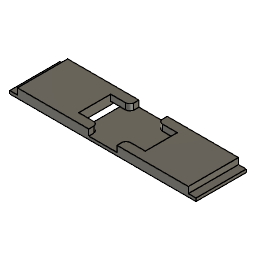
Canal - middle plate v6 (Autodesk Fusion 360 design; units mm, degrees)
Autodesk Fusion 360 part; units mm, degrees
sketch "Esquisse1" plane through (0, 0, 0) normal (0, 0, 1) x (1, 0, 0)
  line L0 (9.4, 40) -> (70, 40)
  line L1 (70, 40) -> (70, 23.65)
  line L2 (70, 23.65) -> (9.4, 23.65)
  line L3 (9.4, 23.65) -> (9.4, 40)
  dimension "d1" = 60.6
  dimension "d2" = 16.35
  constraint horizontal L0
  constraint vertical L1
  constraint horizontal L2
  constraint vertical L3
  measures "d1" distance of L1 L3
  measures "d2" distance of L0 L2
extrude "Extrusion1" add sketch "Esquisse1" along normal blind 3
sketch "Esquisse2" plane through (0, 0, 0) normal (0, 0, -1) x (1, 0, 0)
  line L0 (70, -23.65) -> (9.4, -23.65)
  line L1 (9.4, -23.65) -> (9.4, -40)
  line L2 (9.4, -40) -> (70, -40)
  line L3 (70, -40) -> (70, -23.65)
  line L4 (17.1, -25.55) -> (22.3, -25.55)
  line L5 (22.3, -25.55) -> (22.3, -27.75)
  line L6 (22.3, -27.75) -> (17.1, -27.75)
  line L7 (17.1, -27.75) -> (17.1, -25.55)
  line L8 (19.7, -25.55) -> (19.7, -27.75) construction
  line L9 (39.7, -23.65) -> (39.7, -40) construction
  line L10 (57.1, -25.55) -> (57.1, -27.75)
  line L11 (62.3, -25.55) -> (57.1, -25.55)
  line L12 (62.3, -27.75) -> (62.3, -25.55)
  line L13 (57.1, -27.75) -> (62.3, -27.75)
  line L14 (9.4, -31.825) -> (70, -31.825) construction
  line L15 (17.1, -38.1) -> (22.3, -38.1)
  line L16 (22.3, -38.1) -> (22.3, -35.9)
  line L17 (22.3, -35.9) -> (17.1, -35.9)
  line L18 (17.1, -35.9) -> (17.1, -38.1)
  line L19 (62.3, -38.1) -> (57.1, -38.1)
  line L20 (62.3, -35.9) -> (62.3, -38.1)
  line L21 (57.1, -35.9) -> (62.3, -35.9)
  line L22 (57.1, -38.1) -> (57.1, -35.9)
  dimension "d5" = 20
  dimension "d12" = 5.2
  dimension "d13" = 2.2
  dimension "d14" = 1.9
  constraint horizontal L4
  constraint vertical L5
  constraint horizontal L6
  constraint vertical L7
  constraint midpoint L4 L8.start
  constraint midpoint L6 L8.end
  constraint midpoint L0 L9.start
  constraint midpoint L2 L9.end
  constraint symmetric L4.start L9 L11.start
  constraint symmetric L4.end L9 L10.start
  constraint symmetric L5.end L9 L10.end
  constraint symmetric L6.end L9 L12.start
  constraint midpoint L1 L14.start
  constraint midpoint L3 L14.end
  constraint symmetric L4.start L14 L15.start
  constraint symmetric L4.end L14 L15.end
  constraint symmetric L5.end L14 L16.end
  constraint symmetric L6.end L14 L17.end
  constraint symmetric L10.start L14 L19.end
  constraint symmetric L10.end L14 L21.start
  constraint symmetric L11.start L14 L19.start
  constraint symmetric L12.start L14 L20.start
  measures "d5" distance of L8 L9
  measures "d12" distance of L5 L7
  measures "d13" distance of L4 L6
  measures "d14" distance of L0 L4
extrude "Extrusion2" cut sketch "Esquisse2" against normal blind 2 contours L4 L5 L6 L7 | L10 L11 L12 L13 | L15 L16 L17 L18 | L19 L20 L21 L22
sketch "Esquisse3" plane through (0, 0, 3) normal (0, 0, 1) x (-1, 0, 0)
  line L0 (-9.4, -23.65) -> (-70, -23.65)
  line L1 (-70, -23.65) -> (-70, -40)
  line L2 (-70, -40) -> (-9.4, -40)
  line L3 (-9.4, -40) -> (-9.4, -23.65)
  line L4 (-28.875, -39.65) -> (-50.525, -39.65)
  line L5 (-50.525, -39.65) -> (-50.525, -24)
  line L6 (-50.525, -24) -> (-28.875, -24)
  line L7 (-28.875, -24) -> (-28.875, -39.65)
  line L8 (-9.4, -31.825) -> (-70, -31.825) construction
  line L9 (-39.7, -40) -> (-39.7, -23.65) construction
  line L10 (-50.525, -26.625) -> (-45.775, -26.625)
  line L11 (-44.275, -25.125) -> (-44.275, -24)
  line L12 (-35.125, -24) -> (-35.125, -25.125)
  line L13 (-28.875, -37.025) -> (-33.625, -37.025)
  line L14 (-35.125, -38.525) -> (-35.125, -39.65)
  line L15 (-50.525, -37.025) -> (-45.775, -37.025)
  line L16 (-44.275, -38.525) -> (-44.275, -39.65)
  line L17 (-33.625, -26.625) -> (-28.875, -26.625)
  arc A0 (-45.775, -26.625) -> (-44.275, -25.125) centre (-45.775, -25.125) ccw
  arc A1 (-35.125, -25.125) -> (-33.625, -26.625) centre (-33.625, -25.125) ccw
  arc A2 (-33.625, -37.025) -> (-35.125, -38.525) centre (-33.625, -38.525) ccw
  arc A3 (-44.275, -38.525) -> (-45.775, -37.025) centre (-45.775, -38.525) ccw
  dimension "d8" = 21.65
  dimension "d9" = 15.65
  dimension "d30" = 10.4
  dimension "d31" = 10.4
  dimension "d32" = 9.15
  dimension "d33" = 9.15
  dimension "d34" = 1.5
  constraint horizontal L4
  constraint vertical L5
  constraint horizontal L6
  constraint vertical L7
  constraint midpoint L3 L8.start
  constraint midpoint L1 L8.end
  constraint midpoint L2 L9.start
  constraint midpoint L0 L9.end
  constraint symmetric L5 L7 L9
  constraint symmetric L0 L2 L8
  constraint symmetric L4 L6 L8
  constraint coincident L5 L10.start
  constraint perpendicular L5 L10
  constraint coincident L6 L11.end
  constraint perpendicular L6 L11
  constraint coincident L6 L12.start
  constraint perpendicular L6 L12
  constraint coincident L7 L13.start
  constraint perpendicular L7 L13
  constraint coincident L4 L14.end
  constraint perpendicular L4 L14
  constraint coincident L5 L15.start
  constraint perpendicular L5 L15
  constraint coincident L4 L16.end
  constraint perpendicular L4 L16
  constraint coincident L7 L17.end
  constraint perpendicular L7 L17
  constraint symmetric L8 L13 L17
  constraint symmetric L8 L10 L15
  constraint symmetric L9 L11 L12
  constraint symmetric L9 L14 L16
  constraint tangent L10 A0
  constraint tangent L11 A0
  constraint tangent L12 A1
  constraint tangent L17 A1
  constraint equal A0 A1
  constraint tangent L13 A2
  constraint tangent L14 A2
  constraint equal A0 A2
  constraint tangent L15 A3
  constraint tangent L16 A3
  constraint equal A0 A3
  measures "d8" distance of L5 L7
  measures "d9" distance of L4 L6
  measures "d30" distance of L13 L17
  measures "d31" distance of L10 L15
  measures "d32" distance of L11 L12
  measures "d33" distance of L14 L16
  measures "d34" radius of A0
extrude "Extrusion3" cut sketch "Esquisse3" against normal blind 2 contours L4 L5 L6 L7 L10 L11 L12 L13 L14 L15 L16 L17 A0 A1 A2 A3
sketch "Esquisse4" plane through (0, 0, 1) normal (0, 0, 1) x (-1, 0, 0)
  line L0 (-35.125, -24) -> (-44.275, -24)
  line L1 (-50.525, -26.625) -> (-50.525, -37.025)
  line L2 (-44.275, -39.65) -> (-35.125, -39.65)
  line L3 (-28.875, -37.025) -> (-28.875, -26.625)
  line L4 (-28.875, -26.625) -> (-31.875, -26.625)
  line L5 (-31.875, -26.625) -> (-31.875, -39.65)
  line L6 (-31.875, -39.65) -> (-28.875, -39.65)
  line L7 (-28.875, -39.65) -> (-28.875, -26.625)
  line L8 (-50.525, -37.025) -> (-45.775, -37.025)
  line L9 (-44.275, -38.525) -> (-44.275, -39.65)
  line L10 (-35.125, -39.65) -> (-35.125, -38.525)
  line L11 (-33.625, -37.025) -> (-28.875, -37.025)
  line L12 (-28.875, -26.625) -> (-33.625, -26.625)
  line L13 (-35.125, -25.125) -> (-35.125, -24)
  line L14 (-44.275, -24) -> (-44.275, -25.125)
  line L15 (-45.775, -26.625) -> (-50.525, -26.625)
  arc A0 (-44.275, -38.525) -> (-45.775, -37.025) centre (-45.775, -38.525) ccw
  arc A1 (-33.625, -37.025) -> (-35.125, -38.525) centre (-33.625, -38.525) ccw
  arc A2 (-35.125, -25.125) -> (-33.625, -26.625) centre (-33.625, -25.125) ccw
  arc A3 (-45.775, -26.625) -> (-44.275, -25.125) centre (-45.775, -25.125) ccw
  dimension "d15" = 3
  constraint horizontal L4
  constraint vertical L5
  constraint horizontal L6
  constraint vertical L7
  constraint coincident L2 L5.end
  constraint coincident L3.end L4.start
  measures "d15" distance of L5 L7
extrude "Extrusion4" cut sketch "Esquisse4" against normal blind 3 contours L3 L4 L5 L7 L11 L12 | L5 L6 L7 L11
sketch "Esquisse5" plane through (0, 40, 0) normal (0, 1, 0) x (-1, 0, 0)
  line L0 (-70, 0) -> (-9.4, 0)
  line L1 (-9.4, 0) -> (-9.4, 3)
  line L2 (-9.4, 3) -> (-70, 3)
  line L3 (-70, 3) -> (-70, 0)
  line L4 (-39.7, 3) -> (-39.7, 0) construction
  line L5 (-44.3, 3) -> (-35.1, 3)
  line L6 (-35.1, 3) -> (-35.1, 1)
  line L7 (-35.1, 1) -> (-44.3, 1)
  line L8 (-44.3, 1) -> (-44.3, 3)
  dimension "d18" = 9.2
  dimension "d19" = 2
  constraint midpoint L2 L4.start
  constraint midpoint L0 L4.end
  constraint horizontal L5
  constraint vertical L6
  constraint horizontal L7
  constraint vertical L8
  constraint coincident L2 L5.start
  constraint symmetric L4 L6 L8
  measures "d18" distance of L6 L8
  measures "d19" distance of L5 L7
extrude "Extrusion5" cut sketch "Esquisse5" against normal blind 21 contours L2 L5 L6 L7 L8
sketch "Esquisse6" plane through (0, 0, 3) normal (0, 0, 1) x (-1, 0, 0)
  line L0 (-44.3, -25.3977) -> (-44.3, -23.65)
  line L1 (-44.3, -23.65) -> (-70, -23.65)
  line L2 (-70, -23.65) -> (-70, -40)
  line L3 (-70, -40) -> (-44.3, -40)
  line L4 (-44.3, -40) -> (-44.3, -38.2523)
  line L5 (-50.525, -37.025) -> (-50.525, -26.625)
  line L6 (-70, -40) -> (-67.5, -40)
  line L7 (-67.5, -40) -> (-67.5, -23.65)
  line L8 (-67.5, -23.65) -> (-70, -23.65)
  line L9 (-70, -23.65) -> (-70, -40)
  line L10 (-39.7, -39) -> (-39.7, -18) construction
  line L11 (-9.4, -23.65) -> (-9.4, -40)
  line L12 (-11.9, -23.65) -> (-9.4, -23.65)
  line L13 (-11.9, -40) -> (-11.9, -23.65)
  line L14 (-9.4, -40) -> (-11.9, -40)
  line L15 (-45.775, -37.025) -> (-50.525, -37.025)
  line L16 (-50.525, -26.625) -> (-45.775, -26.625)
  arc A0 (-44.3, -38.2523) -> (-45.775, -37.025) centre (-45.775, -38.525) ccw
  arc A1 (-45.775, -26.625) -> (-44.3, -25.3977) centre (-45.775, -25.125) ccw
  dimension "d22" = 2.5
  dimension "d23" = 30.3
  constraint horizontal L6
  constraint vertical L7
  constraint horizontal L8
  constraint vertical L9
  constraint coincident L1 L7.end
  constraint coincident L2.end L3.start
  constraint parallel L5 L10
  constraint symmetric L2.end L10 L11.end
  constraint symmetric L6.end L10 L13.start
  constraint symmetric L7.end L10 L12.start
  constraint symmetric L1.end L10 L11.start
  measures "d22" distance of L7 L9
  measures "d23" distance of L9 L10
extrude "Extrusion6" cut sketch "Esquisse6" against normal blind 2 contours L1 L2 L3 L6 L7 L8 L9 | L11 L12 L13 L14
